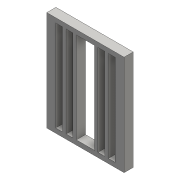
# Autodesk Inventor part: jtd_tack_no_middle_20170113
Saved by Autodesk Inventor 2016 (Build 200138000, 138)
## iProperties
Created: 2016-09-14
Part Number: jtd_tack_no_middle_20170113
Material: Generic
Document SubType Name: Modeling
Designer: Jonathan
Density: 1 g/cm^3
Appearance: Default
Author: Jonathan
Autodesk Inventor part; units mm, degrees
ref_plane "YZ Plane" through (0, 0, 0) normal (1, 0, 0) x (0, 1, 0)
ref_plane "XZ Plane" through (0, 0, 0) normal (0, 1, 0) x (-1, 0, 0)
ref_plane "XY Plane" through (0, 0, 0) normal (0, 0, 1) x (1, 0, 0)
sketch "Sketch1" plane through (0, 0, 0) normal (0, 1, 0) x (-1, 0, 0)
  line L0 (8.5, 11) -> (-8.5, 11)
  line L1 (-8.5, 11) -> (-8.5, -11)
  line L2 (-8.5, -11) -> (8.5, -11)
  line L3 (8.5, -11) -> (8.5, 11)
  line L4 (8.5, 11) -> (-8.5, -11) construction
  line L5 (-8.5, 11) -> (8.5, -11) construction
  point P0 (0, 0)
  dimension "d0" = 17
  dimension "d1" = 22
  constraints: 12 end point, 2 midpoint, 2 parallel, 1 horizontal, 1 perpendicular
  measures "d0" distance of L2.end L1.end
  measures "d1" distance of L0.end L1.end
extrude "Body" add sketch "Sketch1" along normal blind 2
sketch "Sketch3" plane through (0, 2, 0) normal (0, 1, 0) x (1, 0, 0)
  line L0 (8.5, 11) -> (-8.5, 11) projected
  line L1 (0, 11) -> (0, -11)
  line L2 (-8.5, -11) -> (8.5, -11) projected
  line L3 (-2, -10) -> (-0.5, -10)
  line L4 (-0.5, -10) -> (-0.5, 10)
  line L5 (-0.5, 10) -> (-2, 10)
  line L6 (-2, 10) -> (-2, -10)
  line L7 (-2, -10) -> (-0.5, 10) construction
  line L8 (-0.5, -10) -> (-2, 10) construction
  line L9 (-4.25, 10) -> (-2.75, 10)
  line L10 (-2.75, 10) -> (-2.75, -10)
  line L11 (-2.75, -10) -> (-4.25, -10)
  line L12 (-4.25, -10) -> (-4.25, 10)
  line L13 (-4.25, 10) -> (-2.75, -10) construction
  line L14 (-2.75, 10) -> (-4.25, -10) construction
  line L15 (-8.5, 11) -> (-8.5, -11) projected
  line L16 (-8.5, 0) -> (8.5, 0)
  line L17 (-6.55, 10) -> (-5.05, 10)
  line L18 (-5.05, 10) -> (-5.05, -10)
  line L19 (-5.05, -10) -> (-6.55, -10)
  line L20 (-6.55, -10) -> (-6.55, 10)
  line L21 (-6.55, 10) -> (-5.05, -10) construction
  line L22 (-5.05, 10) -> (-6.55, -10) construction
  line L23 (2, -10) -> (0.5, -10)
  line L24 (0.5, -10) -> (0.5, 10)
  line L25 (0.5, 10) -> (2, 10)
  line L26 (2, 10) -> (2, -10)
  line L27 (2, -10) -> (0.5, 10) construction
  line L28 (0.5, -10) -> (2, 10) construction
  line L29 (4.25, 10) -> (2.75, 10)
  line L30 (2.75, 10) -> (2.75, -10)
  line L31 (2.75, -10) -> (4.25, -10)
  line L32 (4.25, -10) -> (4.25, 10)
  line L33 (4.25, 10) -> (2.75, -10) construction
  line L34 (2.75, 10) -> (4.25, -10) construction
  line L35 (6.55, 10) -> (5.05, 10)
  line L36 (5.05, 10) -> (5.05, -10)
  line L37 (5.05, -10) -> (6.55, -10)
  line L38 (6.55, -10) -> (6.55, 10)
  line L39 (6.55, 10) -> (5.05, -10) construction
  line L40 (5.05, 10) -> (6.55, -10) construction
  point P0 (0, 0)
  point P1 (-1.25, 0)
  point P2 (-3.5, 0)
  point P3 (-5.8, 0)
  point P4 (1.25, 0)
  point P5 (3.5, 0)
  point P6 (5.8, 0)
  dimension "d6" = 1.5
  dimension "d7" = 20
  dimension "d9" = 0.5
  dimension "d11" = 2.75
  dimension "d12" = 5.05
  constraints: 76 end point, 15 midpoint, 15 symmetric about line, 6 parallel, 4 equal length, 4 horizontal, 3 perpendicular, 3 other
  measures "d6" distance of L5.end L4.end
  measures "d7" distance of L4.end L3.end
  measures "d9" distance from line of point (0, 0) L4
  measures "d11" distance between parallel lines of L1 L10
  measures "d12" distance between parallel lines of L1 L18
extrude "Rungs" cut sketch "Sketch3" against normal through all contours L36 L35 L38 L16 | L16 L38 L37 L36 | L30 L29 L32 L16 | L16 L32 L31 L30 | L24 L25 L26 L16 | L16 L26 L23 L24 | L16 L6 L5 L4 | L4 L3 L6 L16 | L20 L17 L18 L16 | L16 L18 L19 L20 | L16 L12 L9 L10 | L10 L11 L12 L16
sketch "Sketch4" plane through (0, 2, 0) normal (0, 1, 0) x (1, 0, 0)
  line L0 (0.5, -10) -> (0.5, 10) projected
  line L1 (-2, 10) -> (-0.5, 10) projected
  line L2 (0.5, -10) -> (-0.5, -10)
  line L3 (-0.5, -10) -> (-0.5, 10)
  line L4 (-0.5, 10) -> (0.5, 10)
  line L5 (0.5, 10) -> (0.5, -10)
  point P0 (0, 0)
  constraints: 8 end point, 2 parallel, 1 horizontal, 1 perpendicular
extrude "Remove center rung" cut sketch "Sketch4" against normal through all
body "Solid1"
